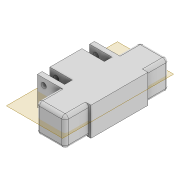
# Autodesk Inventor part: Square_tube_connector
Saved by Autodesk Inventor 2022 (Build 260153000, 153)
## iProperties
Created: 2022-05-02
Part Number: Square_tube_connector
Material: Generic
Document SubType Name: Modeling
Designer: dell
Density: 1 g/cm^3
Appearance: Default
Author: dell
Autodesk Inventor part; units mm, degrees
ref_plane "YZ Plane" through (0, 0, 0) normal (1, 0, 0) x (0, 1, 0)
ref_plane "XZ Plane" through (0, 0, 0) normal (0, 1, 0) x (-1, 0, 0)
ref_plane "XY Plane" through (0, 0, 0) normal (0, 0, 1) x (1, 0, 0)
sketch "Sketch1" plane through (0, 0, 0) normal (0, 1, 0) x (-1, 0, 0)
  line L0 (0, 0) -> (17.9, 0)
  line L1 (17.9, 0) -> (17.9, -64.8)
  line L2 (17.9, -64.8) -> (0, -64.8)
  line L3 (0, -64.8) -> (0, 0)
  line L4 (17.9, -14.6) -> (31.9, -14.6)
  line L5 (31.9, -14.6) -> (31.9, -17.6)
  line L6 (31.9, -17.6) -> (17.9, -17.6)
  line L7 (17.9, -17.6) -> (17.9, -14.6)
  line L8 (17.9, -22.4) -> (31.9, -22.4)
  line L9 (31.9, -22.4) -> (31.9, -42.4)
  line L10 (31.9, -42.4) -> (17.9, -42.4)
  line L11 (17.9, -42.4) -> (17.9, -22.4)
  line L12 (17.9, -47.2) -> (31.9, -47.2)
  line L13 (31.9, -47.2) -> (31.9, -50.2)
  line L14 (31.9, -50.2) -> (17.9, -50.2)
  line L15 (17.9, -50.2) -> (17.9, -47.2)
  line L16 (47.989, -20) -> (-6.1915, -20) construction
  line L17 (47.989, -44.8) -> (-4.845, -44.8) construction
  line L18 (0, -50.2) -> (-1.5, -50.2)
  line L19 (-1.5, -50.2) -> (-1.5, -14.6)
  line L20 (-1.5, -14.6) -> (0, -14.6)
  line L21 (0, -14.6) -> (0, -50.2)
  point P0 (17.9, -42.4)
  point P1 (0, -14.6)
  dimension "d0" = 17.9
  dimension "d2" = 3
  dimension "d4" = 20
  dimension "d5" = 24.8
  dimension "d6" = 2.4
  dimension "d7" = 2.4
  dimension "d8" = 2.4
  dimension "d9" = 2.4
  dimension "d10" = 3
  dimension "d11" = 14
  dimension "d14" = 20
  dimension "d24" = 1.5
  constraints: 44 end point, 10 parallel, 7 horizontal, 6 point on line, 5 perpendicular, 2 collinear
  measures "d0" distance between parallel lines of L3 L1
  measures "d2" distance between parallel lines of L6 L4
  measures "d4" distance between parallel lines of L0 L16
  measures "d5" distance between parallel lines of L17 L16
  measures "d6" distance between parallel lines of L16 L6
  measures "d7" distance between parallel lines of L8 L16
  measures "d8" distance between parallel lines of L17 L10
  measures "d9" distance between parallel lines of L17 L12
  measures "d10" distance between parallel lines of L12 L14
  measures "d11" distance between parallel lines of L1 L5
  measures "d14" distance between parallel lines of L17 L2
  measures "d24" distance between parallel lines of L3 L19
extrude "Extrusion1" add sketch "Sketch1" along normal blind 17.9
fillet "Fillet1" radius 2 16 edges at (-17.9, 8.95, -64.8) (-8.95, 0, -64.8) (0, 8.95, -64.8) (-8.95, 17.9, -64.8) (-8.95, 17.9, 0) (-17.9, 8.95, 0) (-8.95, 0, 0) (0, 8.95, 0) (0, 17.9, -7.3) (0, 17.9, -57.5) (0, 0, -7.3) (0, 0, -57.5) (-17.9, 17.9, -57.5) (-17.9, 0, -57.5) (-17.9, 17.9, -7.3) (-17.9, 0, -7.3)
sketch "Sketch2" plane through (-31.9, 0, -14.6) normal (0, 0, 1) x (1, 0, 0)
  circle A0 centre (4, 13.9) radius 1.6
  circle A1 centre (4, 4) radius 1.6
  line L0 (14, 15.9) -> (14, 2) projected
  line L1 (0, 0) -> (16, 0) projected
  line L2 (0, 17.9) -> (16, 17.9) projected
  point P0 (31.9, 0)
  point P1 (14, 17.8)
  point P2 (14, 0)
  point P3 (12, 0)
  point P4 (12, 17.8)
  point P5 (12.5359, 0)
  point P6 (12.5359, 17.8)
  point P7 (16, 17.9)
  dimension "d16" = 3.2
  dimension "d17" = 3.2
  dimension "d18" = 10
  dimension "d19" = 10
  dimension "d20" = 4
  dimension "d21" = 4
  constraints: 2 centre point, 1 other
  measures "d16" diameter of A0
  measures "d17" diameter of A1
  measures "d18" distance from line of L0 A1.centre
  measures "d19" distance from line of L0 A0.centre
  measures "d20" distance from line of L1 A1.centre
extrude "Extrusion2" cut sketch "Sketch2" against normal blind 100
ref_plane "Work Plane1" through (0, 8.95, 0) normal (0, 1, 0) x (1, 0, 0)
equation "\"d7\" = d6"
equation "\"d8\" = d6"
equation "\"d9\" = d6"
equation "\"d19\" = d18"
body "Solid1"
